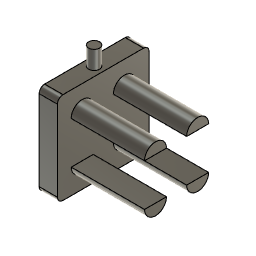
12-garra_completa (Autodesk Fusion 360 archive; units mm, degrees)
design "base_garra"
Autodesk Fusion 360 part; units mm, degrees
sketch "Sketch1" plane through (0, 0, 0) normal (1, 0, 0) x (0, 1, 0)
  circle A0 centre (0, 0) radius 10
  line L0 (25, 25) -> (-25, 25)
  line L1 (-25, 25) -> (-25, -25)
  line L2 (-25, -25) -> (25, -25)
  line L3 (25, -25) -> (25, 25)
  line L4 (11.5, 11.5) -> (-11.5, 11.5) construction
  line L5 (-11.5, 11.5) -> (-11.5, -11.5) construction
  line L6 (-11.5, -11.5) -> (11.5, -11.5) construction
  line L7 (11.5, -11.5) -> (11.5, 11.5) construction
  line L8 (-11.5, 11.5) -> (-11.5, -11.5) construction
  line L9 (11.5, 11.5) -> (11.5, -20) construction
  line L10 (-11.5, 11.5) -> (-11.5, -11.5) construction
  line L11 (5.5, 11.5) -> (5.5, -11.5)
  arc A1 (5.5, -11.5) -> (17.5, -11.5) centre (11.5, -11.5) ccw
  line L12 (17.5, -11.5) -> (17.5, 11.5)
  arc A2 (17.5, 11.5) -> (5.5, 11.5) centre (11.5, 11.5) ccw
  line L13 (11.5, 11.5) -> (11.5, -11.5) construction
  line L14 (-17.5, 11.5) -> (-17.5, -11.5)
  arc A3 (-17.5, -11.5) -> (-5.5, -11.5) centre (-11.5, -11.5) ccw
  line L15 (-5.5, -11.5) -> (-5.5, 11.5)
  arc A4 (-5.5, 11.5) -> (-17.5, 11.5) centre (-11.5, 11.5) ccw
  line L16 (-11.5, 11.5) -> (-11.5, -11.5) construction
  line L17 (-17.5, 11.5) -> (-5.5, 11.5)
  line L18 (-17.5, -11.5) -> (-5.5, -11.5)
  line L19 (17.5, 11.5) -> (5.5, 11.5)
  line L20 (5.5, -11.5) -> (17.5, -11.5)
  dimension "d1" = 20
  dimension "d2" = 25
  dimension "d3" = 11.5
  dimension "d21" = 12
  dimension "d22" = 12
  dimension "d29" = 23
  constraint coincident A0.centre origin
  constraint vertical L3
  constraint horizontal L4
  constraint coincident L5.end L6.start
  constraint perpendicular L4 L8
  constraint coincident L4.end L5.start
  constraint perpendicular L6 L9
  constraint coincident L4.start L7.end
  constraint perpendicular L6 L10
  constraint tangent L11 A1
  constraint tangent A1 L12
  constraint parallel L11 L12
  constraint tangent L12 A2
  constraint tangent L11 A2
  constraint coincident L6.end L7.start
  constraint perpendicular L6 L13
  constraint tangent L14 A3
  constraint tangent A3 L15
  constraint parallel L14 L15
  constraint tangent L15 A4
  constraint tangent L14 A4
  constraint perpendicular L6 L16
  measures "d1" diameter of A0
  measures "d2" distance of A0.centre L3
  measures "d3" distance of A0.centre L7
  measures "d21" diameter of A1
  measures "d22" diameter of A3
  measures "d29" distance of L4.end L5.end
extrude "Extrude1" add sketch "Sketch1" along normal blind 10 contours A0 L11 | A0 L11 L12 L19 L20 | A0 L11 L15 | A0 L15 | A0 L14 L15 L17 L18 | A2 L19 | A1 L20 | A4 L17 | A3 L18 | L0 L1 L2 L3
extrude "Extrude2" add sketch "Sketch1" against normal blind 3 contours A0 L11 | A0 L11 L15 | A0 L15
fillet "Fillet1" radius 3 4 edges at (5, -25, 25) (5, -25, -25) (5, 25, -25) (5, 25, 25)
extrude "Extrude3" add sketch "Sketch1" along normal blind 40 from surface at 10 contours A2 L19 | A1 L20 | A4 L17 | A3 L18
sketch "Sketch4" plane through (0, 0, 11.5) normal (0, 0, -1) x (1, 0, 0)
  line L0 (10, 17.5) -> (10, 5.5)
  line L1 (10, 5.5) -> (50, 5.5)
  line L2 (50, 5.5) -> (50, 17.5)
  line L3 (50, 17.5) -> (10, 17.5)
  line L4 (50, 5.5) -> (10, 17.5) construction
  line L5 (10, 5.5) -> (50, 17.5) construction
  circle A0 centre (30, 11.5) radius 0.5
  dimension "d23" = 1
  constraint coincident L1.end L2.start
  constraint coincident L0.start L3.end
  constraint coincident L0.end L1.start
  constraint coincident L2.end L3.start
  constraint midpoint L4 A0.centre
  measures "d23" diameter of A0
extrude "Extrude6" cut sketch "Sketch4" against normal blind 1 contours A0
sketch "Sketch5" plane through (0, 0, 11.5) normal (0, 0, -1) x (1, 0, 0)
  line L0 (10, -5.5) -> (10, -17.5)
  line L1 (10, -17.5) -> (50, -17.5)
  line L2 (50, -17.5) -> (50, -5.5)
  line L3 (50, -5.5) -> (10, -5.5)
  line L4 (10, -5.5) -> (50, -17.5) construction
  line L5 (10, -17.5) -> (50, -5.5) construction
  circle A0 centre (30, -11.5) radius 0.5
  dimension "d26" = 1
  constraint coincident L0.start L3.end
  constraint coincident L1.end L2.start
  constraint coincident L0.end L1.start
  constraint coincident L2.end L3.start
  constraint midpoint L5 A0.centre
  measures "d26" diameter of A0
extrude "Extrude7" cut sketch "Sketch5" against normal blind 1 contours A0
sketch "Sketch6" plane through (0, 0, 25) normal (0, 0, 1) x (-1, 0, 0)
  line L0 (-10, -22) -> (0, -22)
  line L1 (0, -22) -> (0, 22)
  line L2 (0, 22) -> (-10, 22)
  line L3 (-10, 22) -> (-10, -22)
  line L4 (0, -22) -> (-10, 22) construction
  line L5 (0, 22) -> (-10, -22) construction
  circle A0 centre (-5, 0) radius 3
  dimension "d51" = 6
  constraint coincident L0.end L1.start
  constraint coincident L2.end L3.start
  constraint coincident L1.end L2.start
  constraint coincident L0.start L3.end
  constraint midpoint L4 A0.centre
  measures "d51" diameter of A0
extrude "Extrude8" add sketch "Sketch6" along normal blind 10 contours A0

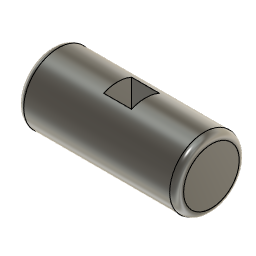
design "conexão_garra_garra"
Autodesk Fusion 360 part; units mm, degrees
sketch "Sketch1" plane through (0, 0, 0) normal (1, 0, 0) x (0, 1, 0)
  circle A0 centre (0, 0) radius 5
  circle A1 centre (0, 0) radius 0.5
  dimension "d1" = 10
  dimension "d2" = 1
  constraint coincident A0.centre A1.centre
  constraint concentric A0 A1
  measures "d1" diameter of A0
  measures "d2" diameter of A1
extrude "Extrude1" add sketch "Sketch1" along normal blind 23 contours A0 | A1
extrude "Extrude2" add sketch "Sketch1" against normal blind 1 contours A1
fillet "Fillet1" radius 1 2 edges at (0, -4.6616, -1.8081) (23, -4.6616, -1.8081)
sketch "Sketch2" plane through (0, 0, 0) normal (0, 0, 1) x (1, 0, 0)
  line L0 (0, 15) -> (0, -10) construction
  line L1 (11.5, 15) -> (11.5, -7) construction
  line L2 (-5, 0) -> (27.3814, 0) construction
  line L3 (9.5, 2) -> (13.5, 2)
  line L4 (13.5, 2) -> (13.5, -2)
  line L5 (13.5, -2) -> (9.5, -2)
  line L6 (9.5, -2) -> (9.5, 2)
  line L7 (9.5, 2) -> (13.5, -2) construction
  line L8 (13.5, 2) -> (9.5, -2) construction
  point P0 (11.5, 0)
  dimension "d9" = 11.5
  dimension "d10" = 4
  dimension "d11" = 4
  constraint vertical L0
  constraint vertical L1
  constraint perpendicular L1 L2
  constraint horizontal L3
  constraint perpendicular L3 L4
  constraint parallel L3 L5
  constraint parallel L4 L6
  constraint coincident L7 P0
  constraint coincident L8 P0
  constraint coincident L1 P0
  constraint coincident L2 P0
  measures "d9" distance of L0 L1
  measures "d10" distance of L4.end L5.end
  measures "d11" distance of L3.end L4.end
extrude "Extrude3" cut sketch "Sketch2" along normal blind 5
